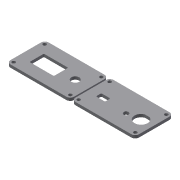
# Autodesk Inventor part: FacePlates 2
Saved by Autodesk Inventor 2015 (Build 190159000, 159)
## iProperties
Created: 2017-06-05
Part Number: FacePlates 2
Material: Generic
Document SubType Name: Modeling
Designer: HAL9000
Density: 1 g/cm^3
Appearance: Default
Author: HAL9000
Autodesk Inventor part; units mm, degrees
ref_plane "YZ Plane" through (0, 0, 0) normal (1, 0, 0) x (0, 1, 0)
ref_plane "XZ Plane" through (0, 0, 0) normal (0, 1, 0) x (-1, 0, 0)
ref_plane "XY Plane" through (0, 0, 0) normal (0, 0, 1) x (1, 0, 0)
sketch "Sketch1" plane through (0, 0, 0) normal (0, 0, 1) x (1, 0, 0)
  line L0 (121.8627, 25) -> (119.4379, 25)
  line L1 (121.8627, 25) -> (124.4458, 25)
  arc A0 (119.4379, 25) -> (124.4458, 25) centre (121.9418, 18.5704) ccw
  circle A1 centre (130.763, 3.7579) radius 1.75
  arc A2 (130.3794, 0) -> (134.3418, 3.9624) centre (130.3794, 3.9624) ccw
  line L2 (134.3418, 35.9156) -> (134.3418, 3.9624)
  arc A3 (134.3418, 35.9156) -> (130.3794, 39.878) centre (130.3794, 35.9156) ccw
  circle A4 centre (130.763, 36.1201) radius 1.75
  circle A5 centre (108.7208, 16.2) radius 2.5
  line L3 (130.3794, 0) -> (71.8832, 0)
  line L4 (130.3794, 39.878) -> (71.8832, 39.878)
  line L5 (71.8832, 39.878) -> (130.3794, 39.878)
  line L6 (130.3794, 39.878) -> (71.8832, 39.878)
  circle A6 centre (96.6208, 18.7) radius 4
  line L7 (87.0208, 20.4) -> (87.0208, 16.8)
  line L8 (87.0208, 16.8) -> (87.0208, 20.4)
  arc A7 (86.0208, 15.8) -> (87.0208, 16.8) centre (86.0208, 16.8) ccw
  arc A8 (86.0208, 15.8) -> (87.0208, 16.8) centre (86.0208, 16.8) ccw
  line L9 (78.5208, 21.4) -> (86.0208, 21.4)
  line L10 (86.0208, 21.4) -> (78.5208, 21.4)
  line L11 (86.0208, 15.8) -> (78.5208, 15.8)
  line L12 (78.5208, 15.8) -> (86.0208, 15.8)
  line L13 (101.1313, 39.878) -> (71.4997, 39.878)
  arc A9 (78.5208, 21.4) -> (77.5208, 20.4) centre (78.5208, 20.4) ccw
  arc A10 (78.5208, 21.4) -> (77.5208, 20.4) centre (78.5208, 20.4) ccw
  circle A11 centre (71.4997, 36.1201) radius 1.75
  arc A12 (77.5208, 16.8) -> (78.5208, 15.8) centre (78.5208, 16.8) ccw
  arc A13 (77.5208, 16.8) -> (78.5208, 15.8) centre (78.5208, 16.8) ccw
  circle A14 centre (71.4997, 3.7579) radius 1.75
  arc A15 (71.8832, 39.878) -> (67.9208, 35.9156) centre (71.8832, 35.9156) ccw
  arc A16 (71.8832, 39.878) -> (67.9208, 35.9156) centre (71.8832, 35.9156) ccw
  arc A17 (67.9208, 3.9624) -> (71.8832, 0) centre (71.8832, 3.9624) ccw
  arc A18 (67.9208, 3.9624) -> (71.8832, 0) centre (71.8832, 3.9624) ccw
  line L14 (77.5208, 16.8) -> (77.5208, 20.4)
  line L15 (77.5208, 20.4) -> (77.5208, 16.8)
  line L16 (3.9624, 0) -> (62.4586, 0)
  line L17 (3.9624, 0) -> (62.4586, 0)
  arc A19 (87.0208, 20.4) -> (86.0208, 21.4) centre (86.0208, 20.4) ccw
  arc A20 (87.0208, 20.4) -> (86.0208, 21.4) centre (86.0208, 20.4) ccw
  line L18 (37.084, 13.192) -> (37.084, 26.192)
  arc A21 (66.421, 35.9156) -> (62.4586, 39.878) centre (62.4586, 35.9156) ccw
  arc A22 (62.4586, 0) -> (66.421, 3.9624) centre (62.4586, 3.9624) ccw
  circle A23 centre (62.8421, 3.7579) radius 1.75
  circle A24 centre (51.4985, 20.192) radius 4.1
  line L19 (37.084, 26.192) -> (37.084, 13.192)
  arc A25 (36.084, 12.192) -> (37.084, 13.192) centre (36.084, 13.192) ccw
  arc A26 (37.084, 26.192) -> (36.084, 27.192) centre (36.084, 26.192) ccw
  line L20 (67.9208, 35.9156) -> (67.9208, 3.9624)
  line L21 (67.9208, 35.9156) -> (67.9208, 3.9624)
  line L22 (67.9208, 3.9624) -> (67.9208, 35.9156)
  line L23 (67.9208, 19.939) -> (67.9208, 36.1201)
  circle A27 centre (62.8421, 36.1201) radius 1.75
  line L24 (66.421, 3.9624) -> (66.421, 35.9156)
  line L25 (36.084, 27.192) -> (12.684, 27.192)
  arc A28 (3.9624, 39.878) -> (0, 35.9156) centre (3.9624, 35.9156) ccw
  arc A29 (3.9624, 39.878) -> (0, 35.9156) centre (3.9624, 35.9156) ccw
  line L26 (62.4586, 39.878) -> (3.9624, 39.878)
  line L27 (62.4586, 39.878) -> (3.9624, 39.878)
  line L28 (12.684, 12.192) -> (36.084, 12.192)
  arc A30 (0, 3.9624) -> (3.9624, 0) centre (3.9624, 3.9624) ccw
  circle A31 centre (3.5789, 3.7579) radius 1.75
  arc A32 (11.684, 13.192) -> (12.684, 12.192) centre (12.684, 13.192) ccw
  line L29 (11.684, 26.192) -> (11.684, 13.192)
  arc A33 (12.684, 27.192) -> (11.684, 26.192) centre (12.684, 26.192) ccw
  line L30 (0, 35.9156) -> (0, 3.9624)
  line L31 (0, 35.9156) -> (0, 3.9624)
  circle A34 centre (3.5789, 36.1201) radius 1.75
  arc A35 (0, 3.9624) -> (3.9624, 0) centre (3.9624, 3.9624) ccw
  point P0 (0, 0)
  dimension "d2" = 28.7
  constraints: 64 end point, 50 point on circle, 36 centre point, 6 midpoint, 2 point on line
  measures "d2" distance from line of L20 A6.centre
extrude "Extrusion1" add sketch "Sketch1" along normal blind 3
sketch "Sketch2" plane through (0, 0, 3) normal (0, 0, 1) x (1, 0, 0)
  arc A0 (119.4379, 25) -> (124.4458, 25) centre (121.9418, 18.5704) ccw projected
  line L0 (119.4379, 25) -> (124.4458, 25) projected
  line L1 (87.0208, 20.4) -> (87.0208, 16.8) projected
  arc A1 (86.0208, 15.8) -> (87.0208, 16.8) centre (86.0208, 16.8) ccw projected
  line L2 (86.0208, 15.8) -> (78.5208, 15.8) projected
  arc A2 (77.5208, 16.8) -> (78.5208, 15.8) centre (78.5208, 16.8) ccw projected
  line L3 (77.5208, 16.8) -> (77.5208, 20.4) projected
  arc A3 (78.5208, 21.4) -> (77.5208, 20.4) centre (78.5208, 20.4) ccw projected
  line L4 (78.5208, 21.4) -> (86.0208, 21.4) projected
  arc A4 (87.0208, 20.4) -> (86.0208, 21.4) centre (86.0208, 20.4) ccw projected
  circle A5 centre (96.6208, 18.7) radius 4 projected
  circle A6 centre (108.7208, 16.2) radius 2.5 projected
  circle A7 centre (71.4997, 3.7579) radius 1.75 projected
  circle A8 centre (71.4997, 36.1201) radius 1.75 projected
  circle A9 centre (130.763, 36.1201) radius 1.75 projected
  circle A10 centre (130.763, 3.7579) radius 1.75 projected
  arc A11 (130.3794, 0) -> (134.3418, 3.9624) centre (130.3794, 3.9624) ccw projected
  line L5 (134.3418, 3.9624) -> (134.3418, 35.9156) projected
  arc A12 (134.3418, 35.9156) -> (130.3794, 39.878) centre (130.3794, 35.9156) ccw projected
  line L6 (130.3794, 39.878) -> (71.8832, 39.878) projected
  arc A13 (71.8832, 39.878) -> (67.9208, 35.9156) centre (71.8832, 35.9156) ccw projected
  line L7 (67.9208, 35.9156) -> (67.9208, 3.9624) projected
  arc A14 (67.9208, 3.9624) -> (71.8832, 0) centre (71.8832, 3.9624) ccw projected
  line L8 (71.8832, 0) -> (130.3794, 0) projected
  point P0 (0, 0)
extrude "Extrusion2" add sketch "Sketch2" against normal blind 3 contours A5
body "Solid1"
